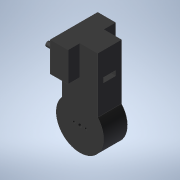
# Autodesk Inventor part: EndConnector
Saved by Autodesk Inventor 2022 (Build 260153000, 153)
## iProperties
Created: 2022-02-04
Part Number: EndConnector
Material: Generic
Document SubType Name: Modeling
Designer: Alexa
Density: 1 g/cm^3
Appearance: Default
Author: Alexa
Autodesk Inventor part; units mm, degrees
ref_plane "YZ Plane" through (0, 0, 0) normal (1, 0, 0) x (0, 1, 0)
ref_plane "XZ Plane" through (0, 0, 0) normal (0, 1, 0) x (-1, 0, 0)
ref_plane "XY Plane" through (0, 0, 0) normal (0, 0, 1) x (1, 0, 0)
sketch "Sketch1" plane through (0, 0, 0) normal (0, 0, 1) x (1, 0, 0)
  circle A0 centre (0, 0) radius 10
  circle A1 centre (0, 0) radius 20
  line L0 (-15, 0) -> (15, 0)
  line L1 (15, 0) -> (15, 50)
  line L2 (15, 50) -> (-15, 50)
  line L3 (-15, 50) -> (-15, 0)
  point P0 (-15, 13.2288)
  point P1 (15, 13.2288)
  dimension "d0" = 20
  dimension "d1" = 40
  dimension "d2" = 30
  dimension "d3" = 50
  constraints: 8 end point, 2 centre point, 2 coincident, 2 parallel, 1 horizontal, 1 perpendicular
  measures "d0" diameter of A0
  measures "d1" diameter of A1
  measures "d2" distance of L2.end L1.end
  measures "d3" distance of L1.end L0.end
extrude "Extrusion1" add sketch "Sketch1" along normal blind 20
sketch "Sketch2" plane through (0, 0, 20) normal (0, 0, 1) x (1, 0, 0)
  circle A0 centre (0, 0) radius 10
  dimension "d6" = 20
  constraints: 1 centre point, 1 coincident
  measures "d6" diameter of A0
extrude "Extrusion2" cut sketch "Sketch2" against normal blind 15
sketch "Sketch4" plane through (-15, 13.2288, 0) normal (-1, 0, 0) x (0, 0, 1)
  line L0 (0, 36.7712) -> (20, 36.7712) projected
  line L1 (0, 0) -> (0, 36.7712) projected
  line L2 (20, 36.7712) -> (0, 36.7712)
  line L3 (0, 36.7712) -> (0, 0)
  line L4 (0, 0) -> (20, 0)
  line L5 (20, 0) -> (20, 36.7712)
  line L6 (0, 0) -> (20, 0) projected
  line L7 (20, 36.7712) -> (10, 36.7712)
  line L8 (10, 36.7712) -> (10, 0)
  line L9 (10, 0) -> (20, 0)
  line L10 (20, 0) -> (20, 36.7712)
  line L11 (10, 0) -> (16, 0)
  line L12 (16, 0) -> (16, 25)
  line L13 (16, 25) -> (10, 25)
  line L14 (10, 25) -> (10, 0)
  line L15 (10, 25) -> (4, 25)
  line L16 (4, 25) -> (4, 0)
  line L17 (4, 0) -> (10, 0)
  line L18 (10, 0) -> (10, 25)
  line L19 (4, 25) -> (16, 25)
  line L20 (16, 25) -> (16, 30.0005)
  line L21 (16, 30.0005) -> (4, 30.0005)
  line L22 (4, 30.0005) -> (4, 25)
  line L23 (4, 30.0005) -> (16, 30.0005)
  line L24 (16, 30.0005) -> (16, 7.0005)
  line L25 (16, 7.0005) -> (4, 7.0005)
  line L26 (4, 7.0005) -> (4, 30.0005)
  line L27 (10, 7.0005) -> (16, 7.0005)
  line L28 (16, 7.0005) -> (16, 0)
  line L29 (16, 0) -> (10, 0)
  line L30 (10, 0) -> (10, 7.0005)
  point P0 (0, -13.2288)
  dimension "d13" = 6
  dimension "d14" = 25
  dimension "d15" = 6
  dimension "d16" = 23
  constraints: 56 end point, 14 parallel, 7 horizontal, 7 perpendicular, 3 point on line, 2 midpoint
  measures "d13" distance of L13.end L12.end
  measures "d14" distance of L12.end L11.end
  measures "d15" distance of L17.end L16.end
  measures "d16" distance of L23.end L24.end
extrude "Extrusion3" cut sketch "Sketch4" against normal blind 23 contours L21 L20 L13 L8 | L8 L15 L22 L21 | L13 L12 L25 L8 | L8 L25 L16 L15
sketch "Sketch6" plane through (-15, 13.2288, 0) normal (-1, 0, 0) x (0, 0, 1)
  line L0 (4, 7.0005) -> (4, 30.0005) projected
  line L1 (4, 7.0005) -> (16, 7.0005)
  line L2 (16, 7.0005) -> (16, 2.2005)
  line L3 (16, 2.2005) -> (4, 2.2005)
  line L4 (4, 2.2005) -> (4, 7.0005)
  line L5 (4, 30.0005) -> (16, 30.0005)
  line L6 (16, 30.0005) -> (16, 34.8005)
  line L7 (16, 34.8005) -> (4, 34.8005)
  line L8 (4, 34.8005) -> (4, 30.0005)
  point P0 (0, -13.2288)
  dimension "d19" = 12
  dimension "d20" = 4.8
  dimension "d21" = 4.8
  constraints: 16 end point, 4 parallel, 2 horizontal, 2 perpendicular, 1 point on line
  measures "d19" distance of L2.end L3.end
  measures "d20" distance of L1.end L2.end
  measures "d21" distance of L6.end L5.end
extrude "Extrusion4" cut sketch "Sketch6" against normal blind 16
sketch "Sketch7" plane through (1, 13.2288, 0) normal (-1, 0, 0) x (0, 0, 1)
  line L0 (4, 30.0005) -> (16, 30.0005) projected
  line L1 (4, 30.0005) -> (10, 30.0005)
  line L2 (10, 30.0005) -> (10, 32.5005)
  line L3 (10, 32.5005) -> (4, 32.5005)
  line L4 (4, 32.5005) -> (4, 30.0005)
  circle A0 centre (10, 32.5005) radius 0.75
  line L5 (16, 7.0005) -> (4, 7.0005) projected
  line L6 (16, 7.0005) -> (16, 2.2005) projected
  line L7 (4, 7.0005) -> (16, 7.0005)
  line L8 (16, 7.0005) -> (16, 4.5005)
  line L9 (16, 4.5005) -> (4, 4.5005)
  line L10 (4, 4.5005) -> (4, 7.0005)
  line L11 (10, 4.5005) -> (4, 4.5005)
  line L12 (4, 4.5005) -> (4, 7.0005)
  line L13 (4, 7.0005) -> (10, 7.0005)
  line L14 (10, 7.0005) -> (10, 4.5005)
  circle A1 centre (10, 4.5005) radius 0.75
  point P0 (0, -13.2288)
  dimension "d24" = 2.5
  dimension "d25" = 1.5
  dimension "d26" = 2.5
  dimension "d27" = 1.5
  constraints: 24 end point, 6 parallel, 3 horizontal, 3 perpendicular, 2 centre point, 2 coincident, 1 midpoint, 1 point on line
  measures "d24" distance of L2.end L1.end
  measures "d25" diameter of A0
  measures "d26" distance of L7.end L8.end
  measures "d27" diameter of A1
extrude "Extrusion5" cut sketch "Sketch7" against normal blind 8 contours A0 L3 L2 | L2 L3 A0 | A1 L9 L14 | L14 L9 A1 | A1 L9
sketch "Sketch8" plane through (15, 13.2288, 0) normal (1, 0, 0) x (0, 0, -1)
  line L0 (0, 36.7712) -> (0, 0) projected
  line L1 (-20, 36.7712) -> (-20, 0) projected
  line L2 (0, 36.7712) -> (-20, 36.7712)
  line L3 (-20, 36.7712) -> (-20, 26.7712)
  line L4 (-20, 26.7712) -> (0, 26.7712)
  line L5 (0, 26.7712) -> (0, 36.7712)
  line L6 (0, 26.7712) -> (-20, 26.7712)
  line L7 (-20, 26.7712) -> (-20, 18.7712)
  line L8 (-20, 18.7712) -> (0, 18.7712)
  line L9 (0, 18.7712) -> (0, 26.7712)
  line L10 (0, 26.7712) -> (-10, 26.7712)
  line L11 (-10, 26.7712) -> (-10, 18.7712)
  line L12 (-10, 18.7712) -> (0, 18.7712)
  line L13 (0, 18.7712) -> (0, 26.7712)
  line L14 (-10, 26.7712) -> (-5, 26.7712)
  line L15 (-5, 26.7712) -> (-5, 22.7712)
  line L16 (-5, 22.7712) -> (-10, 22.7712)
  line L17 (-10, 22.7712) -> (-10, 26.7712)
  line L18 (-10, 22.7712) -> (-15, 22.7712)
  line L19 (-15, 22.7712) -> (-15, 26.7712)
  line L20 (-15, 26.7712) -> (-10, 26.7712)
  line L21 (-10, 26.7712) -> (-10, 22.7712)
  point P0 (0, -13.2288)
  dimension "d30" = 10
  dimension "d31" = 8
  dimension "d32" = 5
  dimension "d33" = 5
  constraints: 40 end point, 10 parallel, 5 horizontal, 5 perpendicular, 3 point on line, 1 midpoint
  measures "d30" distance of L3.end L2.end
  measures "d31" distance of L7.end L6.end
  measures "d32" distance of L15.end L16.end
  measures "d33" distance of L19.end L20.end
extrude "Extrusion6" cut sketch "Sketch8" against normal blind 15.8125 contours L15 L16 L11 L4 | L11 L18 L19 L4
sketch "Sketch9" plane through (0, 0, 5) normal (0, 0, 1) x (1, 0, 0)
  circle A0 centre (0, 0) radius 1
  circle A1 centre (7, 0) radius 1.5
  circle A2 centre (0, 0) radius 1.5
  circle A3 centre (-7, 0) radius 1.5
  dimension "d36" = 2
  dimension "d37" = 3
  dimension "d38" = 3
  dimension "d39" = 3
  constraints: 4 centre point, 2 coincident
  measures "d36" diameter of A0
  measures "d37" diameter of A1
  measures "d38" diameter of A2
  measures "d39" diameter of A3
extrude "Extrusion7" cut sketch "Sketch9" against normal blind 8 contours A0 | A1 | A2 | A3
sketch "Sketch10" plane through (-15, 50, 0) normal (0, 1, 0) x (1, 0, 0)
  line L0 (0, 0) -> (0, -20) projected
  line L1 (0, 0) -> (29.4792, 0)
  line L2 (29.4792, 0) -> (29.4792, -20)
  line L3 (29.4792, -20) -> (0, -20)
  line L4 (0, -20) -> (0, 0)
  point P0 (15, 0)
  constraints: 8 end point, 2 parallel, 1 horizontal, 1 perpendicular
extrude "Extrusion8" add sketch "Sketch10" along normal blind 10
sketch "Sketch11" plane through (0, 0, 0) normal (0, 0, -1) x (-1, 0, 0)
  line L0 (15, 13.2288) -> (15, 60) projected
  line L1 (-15, 13.2288) -> (-15, 50) projected
  line L2 (15, 60) -> (-15, 60)
  line L3 (-15, 60) -> (-15, 45)
  line L4 (-15, 45) -> (15, 45)
  line L5 (15, 45) -> (15, 60)
  line L6 (15, 45) -> (-15, 45)
  line L7 (-15, 45) -> (-15, 35)
  line L8 (-15, 35) -> (15, 35)
  line L9 (15, 35) -> (15, 45)
  point P0 (0, 0)
  dimension "d47" = 15
  dimension "d48" = 10
  constraints: 16 end point, 4 parallel, 2 horizontal, 2 perpendicular, 2 point on line
  measures "d47" distance of L3.end L2.end
  measures "d48" distance of L7.end L6.end
sketch "Sketch12" plane through (14.4792, 50, 20) normal (1, 0, 0) x (0, 0, -1)
  line L0 (20, 0) -> (20, 10) projected
  line L1 (0, 0) -> (20, 0)
  line L2 (20, 0) -> (20, 10)
  line L3 (20, 10) -> (0, 10)
  line L4 (0, 10) -> (0, 0)
  point P0 (20, -50)
  constraints: 8 end point, 2 parallel, 1 horizontal, 1 perpendicular
extrude "Extrusion9" cut sketch "Sketch12" against normal blind 59.6125
sketch "Sketch13" plane through (-15, 50, 0) normal (0, 1, 0) x (1, 0, 0)
  line L0 (30, 0) -> (30, -20) projected
  line L1 (0, 0) -> (30, 0)
  line L2 (30, 0) -> (30, -20)
  line L3 (30, -20) -> (0, -20)
  line L4 (0, -20) -> (0, 0)
  point P0 (15, 0)
  constraints: 8 end point, 2 parallel, 1 horizontal, 1 perpendicular
extrude "Extrusion10" add sketch "Sketch13" along normal blind 10
extrude "Extrusion11" add sketch "Sketch11" along normal blind 10
sketch "Sketch15" plane through (0, 0, 20) normal (0, 0, 1) x (1, 0, 0)
  line L0 (-15, 60) -> (15, 60) projected
  line L1 (-15, 60) -> (0, 60)
  line L2 (0, 60) -> (0, 35)
  line L3 (0, 35) -> (-15, 35)
  line L4 (-15, 35) -> (-15, 60)
  point P0 (0, 0)
  dimension "d56" = 25
  constraints: 8 end point, 2 parallel, 1 horizontal, 1 perpendicular
  measures "d56" distance of L1.end L2.end
extrude "Extrusion12" add sketch "Sketch15" along normal blind 10
sketch "Sketch16" plane through (0, 0, -10) normal (0, 0, -1) x (-1, 0, 0)
  line L0 (-15, 13.2288) -> (-15, 60) projected
  line L1 (0, 35) -> (15, 35) projected
  line L2 (-15, 60) -> (0, 60)
  line L3 (0, 60) -> (0, 35)
  line L4 (0, 35) -> (-15, 35)
  line L5 (-15, 35) -> (-15, 60)
  point P0 (0, 0)
  constraints: 8 end point, 2 parallel, 1 horizontal, 1 perpendicular
extrude "Extrusion13" cut sketch "Sketch16" against normal blind 10
sketch "Sketch17" plane through (-15, 13.2288, 0) normal (-1, 0, 0) x (0, 0, 1)
  line L0 (0, 0) -> (0, 46.7712) projected
  line L1 (0, 46.7712) -> (10, 46.7712)
  line L2 (10, 46.7712) -> (10, 23.4712)
  line L3 (10, 23.4712) -> (0, 23.4712)
  line L4 (0, 23.4712) -> (0, 46.7712)
  circle A0 centre (10, 23.4712) radius 10
  line L5 (20, 46.7712) -> (30, 46.7712) projected
  line L6 (20, 0) -> (20, 46.7712) projected
  line L7 (30, 46.7712) -> (20, 46.7712)
  line L8 (20, 46.7712) -> (20, 36.7712)
  line L9 (20, 36.7712) -> (30, 36.7712)
  line L10 (30, 36.7712) -> (30, 46.7712)
  line L11 (30, 46.7712) -> (24, 46.7712)
  line L12 (24, 46.7712) -> (24, 36.7712)
  line L13 (24, 36.7712) -> (30, 36.7712)
  line L14 (30, 36.7712) -> (30, 46.7712)
  circle A1 centre (24, 36.7712) radius 2
  line L15 (30, 46.7712) -> (-10, 46.7712) projected
  line L16 (-10, 46.7712) -> (-4, 46.7712)
  line L17 (-4, 46.7712) -> (-4, 36.7712)
  line L18 (-4, 36.7712) -> (-10, 36.7712)
  line L19 (-10, 36.7712) -> (-10, 46.7712)
  circle A2 centre (-4, 36.7712) radius 2
  point P0 (0, -13.2288)
  dimension "d61" = 23.3
  dimension "d62" = 20
  dimension "d63" = 10
  dimension "d64" = 6
  dimension "d65" = 4
  dimension "d66" = 6
  dimension "d67" = 4
  constraints: 32 end point, 8 parallel, 4 horizontal, 4 perpendicular, 3 centre point, 3 coincident, 2 point on line
  measures "d61" distance of L1.end L2.end
  measures "d62" diameter of A0
  measures "d63" distance of L8.end L7.end
  measures "d64" distance of L13.end L12.end
  measures "d65" diameter of A1
  measures "d66" distance of L17.end L18.end
  measures "d67" diameter of A2
extrude "Extrusion14" add sketch "Sketch17" along normal blind 8 contours A2 L18 L17 | L17 L18 A2 | A1 L12 L9 | L9 A1 | L12 A1 L9
sketch "Sketch18" plane through (0, 0, 20) normal (0, 0, 1) x (1, 0, 0)
  circle A0 centre (0, 0) radius 10
  constraints: 1 centre point, 1 coincident
extrude "Extrusion15" add sketch "Sketch18" against normal blind 16
sketch "Sketch19" plane through (0, 0, 0) normal (0, 0, -1) x (-1, 0, 0)
  circle A0 centre (0, 0) radius 1.5 projected
  circle A1 centre (0, 0) radius 10
  dimension "d72" = 20
  constraints: 1 centre point, 1 coincident
  measures "d72" diameter of A1
extrude "Extrusion16" cut sketch "Sketch19" against normal blind 16
sketch "Sketch20" plane through (0, 0, 4) normal (0, 0, -1) x (-1, 0, 0)
  circle A0 centre (0, 0) radius 1.5 projected
  circle A1 centre (0, 0) radius 1.5
  constraints: 1 centre point, 1 coincident
extrude "Extrusion17" cut sketch "Sketch20" against normal blind 30.0375
sketch "Sketch21" plane through (0, 0, 16) normal (0, 0, -1) x (-1, 0, 0)
  circle A0 centre (5, 0) radius 1
  circle A1 centre (-5, 0) radius 1
  point P0 (0, 0)
  dimension "d77" = 2
  dimension "d78" = 2
  constraints: 2 centre point
  measures "d77" diameter of A0
  measures "d78" diameter of A1
extrude "Extrusion18" cut sketch "Sketch21" against normal blind 138.2375
chamfer "Chamfer2" distance 8 angle 45 1 edges at (10, 0, 0)
body "Solid1"
